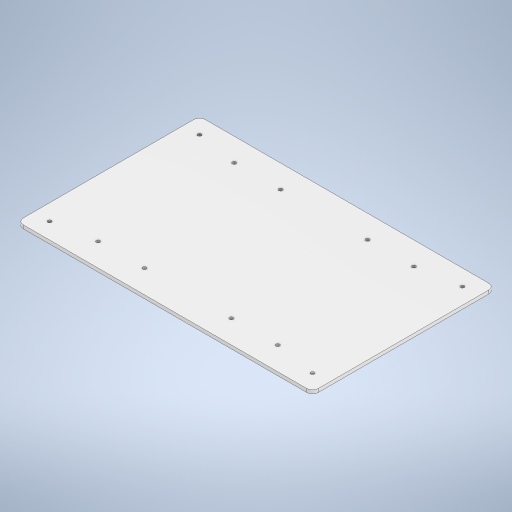
# Autodesk Inventor part: BP_BOX-Under
Saved by Autodesk Inventor 2024.3 (Build 283343000, 343)
## iProperties
Created: 2025-04-29
Part Number: BP_BOX-Under
Material: アセタール樹脂、白
Document SubType Name: Modeling
Designer: ngt-a
Density: 1.425 g/cm^3
Appearance: 滑らか - 白
Mass: 180.144 g
Surface Area: 870.17 cm^2
Volume: 126.417 cm^3
Author: ngt-a
Autodesk Inventor part; units mm, degrees
ref_plane "YZ Plane" through (0, 0, 0) normal (1, 0, 0) x (0, 1, 0)
ref_plane "XZ Plane" through (0, 0, 0) normal (0, 1, 0) x (-1, 0, 0)
ref_plane "XY Plane" through (0, 0, 0) normal (0, 0, 1) x (1, 0, 0)
sketch "スケッチ1" plane through (0, 0, 0) normal (0, 1, 0) x (-1, 0, 0)
  line L0 (130, 81) -> (-130, 81)
  line L1 (-130, 81) -> (-130, -81)
  line L2 (-130, -81) -> (130, -81)
  line L3 (130, -81) -> (130, 81)
  line L4 (130, 81) -> (-130, -81) construction
  line L5 (-130, 81) -> (130, -81) construction
  point P0 (0, 0)
  dimension "d0" = 260
  dimension "d1" = 162
  constraints: 12 end point, 2 midpoint, 2 parallel, 1 horizontal, 1 perpendicular
  measures "d0" distance of L1.end L2.end
  measures "d1" distance of L2.end L0.start
extrude "押し出し1" add sketch "スケッチ1" along normal blind 3
sketch "スケッチ7" plane through (0, 3, 0) normal (0, 1, 0) x (1, 0, 0)
  line L0 (-130, 81) -> (-130, -81) projected
  line L1 (130, -81) -> (130, 81) projected
  line L2 (130, 81) -> (-130, 81) projected
  point P0 (0, 0)
  point P1 (-116, 67)
  point P2 (112, 67)
  point P3 (112, -63)
  point P4 (-116, -63)
  dimension "d23" = 14
  dimension "d25" = 130
  dimension "d26" = 130
  dimension "d27" = 14
  dimension "d29" = 14
  dimension "d38" = 228
  dimension "d39" = 228
  dimension "d40" = 14
  measures "d23" distance from line of L0 point (-116, 67)
  measures "d25" distance of point (112, -63) point (112, 67)
  measures "d26" distance of point (-116, -63) point (-116, 67)
  measures "d27" distance from line of L0 point (-116, -63)
  measures "d29" distance from line of L2 point (-116, 67)
  measures "d38" distance of point (-116, -63) point (112, -63)
  measures "d39" distance of point (-116, 67) point (112, 67)
  measures "d40" distance from line of L2 point (112, 67)
hole "穴1" at (-116, 3, -67) at (112, 3, -67) at (112, 3, 63) at (-116, 3, 63) direction (0, -1, 0) diameter 3.2 depth 8
sketch "スケッチ8" plane through (0, 3, 0) normal (0, 1, 0) x (1, 0, 0)
  line L0 (130, 81) -> (-130, 81) projected
  line L1 (-130, 81) -> (126, 81)
  line L2 (126, 81) -> (126, -77)
  line L3 (126, -77) -> (-130, -77)
  line L4 (-130, -77) -> (-130, 81)
  circle A0 centre (-116, 67) radius 1.6 projected
  circle A1 centre (112, 67) radius 1.6 projected
  circle A2 centre (-116, -63) radius 1.6 projected
  circle A3 centre (-116, -63) radius 1.6 projected
  circle A4 centre (112, -63) radius 1.6 projected
  circle A5 centre (112, 67) radius 1.6 projected
  circle A6 centre (-116, 67) radius 1.6 projected
  line L5 (130, -81) -> (130, 81) projected
  line L6 (130, 81) -> (-130, 81) projected
  line L7 (-130, 81) -> (-130, -81) projected
  line L8 (-130, -81) -> (130, -81) projected
  point P0 (0, 0)
  dimension "d41" = 14
  dimension "d42" = 14
  dimension "d43" = 14
  constraints: 8 end point, 2 parallel, 1 horizontal, 1 perpendicular
  measures "d41" distance from line of L4 A0.centre
  measures "d42" distance from line of L2 A1.centre
  measures "d43" distance from line of L3 A2.centre
extrude "押し出し4" cut sketch "スケッチ8" against normal blind 10 contours L5 L8 L7 L3 L2 L0
fillet "フィレット1" radius 5 4 edges at (-130, 1.5, -81) (-130, 1.5, 77) (126, 1.5, -81) (126, 1.5, 77)
sketch "スケッチ9" plane through (0, 3, 0) normal (0, 1, 0) x (1, 0, 0)
  line L0 (-130, 76) -> (-130, -72) projected
  line L1 (-89.9, 81) -> (-69.9, 81)
  line L2 (-69.8, 81) -> (-49.8, 81)
  line L3 (-49.7, 81) -> (-29.7, 81)
  line L4 (-29.7, -77) -> (-49.7, -77)
  line L5 (0, 0) -> (0, 16.1014)
  circle A0 centre (-116, 67) radius 1.6 projected
  line L6 (126, -72) -> (126, 76) projected
  line L7 (121, 81) -> (-125, 81) projected
  line L8 (-125, -77) -> (121, -77) projected
  line L9 (-69.8, 81) -> (-49.8, 81)
  line L10 (-49.8, 81) -> (-49.8, -77)
  line L11 (-49.8, -77) -> (-69.8, -77)
  line L12 (-69.8, -77) -> (-69.8, 81)
  line L13 (45.8, 81) -> (65.8, 81)
  line L14 (65.8, 81) -> (65.8, -77)
  line L15 (65.8, -77) -> (45.8, -77)
  line L16 (45.8, -77) -> (45.8, 81)
  line L17 (-69.9, 81) -> (-89.9, 81)
  line L18 (-89.9, 81) -> (-89.9, -77)
  line L19 (-89.9, -77) -> (-69.9, -77)
  line L20 (-69.9, -77) -> (-69.9, 81)
  line L21 (121, 81) -> (-125, 81) projected
  line L22 (-49.7, 81) -> (-29.7, 81)
  line L23 (-29.7, 81) -> (-29.7, -77)
  line L24 (-29.7, -77) -> (-49.7, -77)
  line L25 (-49.7, -77) -> (-49.7, 81)
  point P0 (-79.9, 61)
  point P1 (-39.7, 61)
  point P2 (-79.9, -57)
  point P3 (-39.7, -57)
  point P4 (75.9, 61)
  point P5 (35.7, 61)
  point P6 (75.9, -57)
  point P7 (35.7, -57)
  point P8 (-79.9, 81)
  point P9 (-59.8, 61)
  point P10 (55.8, 61)
  point P11 (55.8, -57)
  point P12 (-59.8, -57)
  dimension "d77" = 118
  dimension "d114" = 20
  dimension "d115" = 20
  dimension "d116" = 20
  dimension "d117" = 20
  dimension "d118" = 20
  dimension "d119" = 20
  dimension "d120" = 20
  dimension "d121" = 20
  dimension "d122" = 70.2
  dimension "d123" = 70.2
  dimension "d124" = 20
  dimension "d125" = 70.2
  dimension "d126" = 70.2
  dimension "d127" = 10
  dimension "d128" = 10
  dimension "d129" = 10
  dimension "d130" = 10
  dimension "d131" = 10
  dimension "d132" = 0.1
  dimension "d133" = 50.1
  dimension "d134" = 50.1
  dimension "d135" = 10
  dimension "d136" = 118
  dimension "d137" = 50.1
  dimension "d138" = 10
  dimension "d139" = 0.1
  dimension "d140" = 10
  dimension "d141" = 90.3
  dimension "d142" = 90.3
  dimension "d143" = 90.3
  dimension "d144" = 90.3
  dimension "d145" = 50.1
  constraints: 42 end point, 9 parallel, 7 horizontal, 4 perpendicular, 4 point on line, 1 midpoint, 1 vertical, 5 other
  measures "d77" distance of point (35.7, 61) point (35.7, -57)
  measures "d114" distance of point (-79.9, 81) point (-79.9, 61)
  measures "d116" distance from line of L8 point (-79.9, -57)
  measures "d117" distance from line of L8 point (-39.7, -57)
  measures "d118" distance from line of L8 point (35.7, -57)
  measures "d119" distance from line of L8 point (75.9, -57)
  measures "d122" distance from line of L0 point (-59.8, 61)
  measures "d123" distance from line of L6 point (55.8, 61)
  measures "d124" distance from line of L11 point (-59.8, -57)
  measures "d125" distance from line of L0 point (-59.8, -57)
  measures "d126" distance from line of L6 point (55.8, -57)
  measures "d127" distance from line of L10 point (-59.8, 61)
  measures "d128" distance from line of L12 point (-59.8, 61)
  measures "d129" distance from line of L14 point (55.8, 61)
  measures "d130" distance from line of L16 point (55.8, 61)
  measures "d131" distance from line of L20 point (-79.9, 61)
  measures "d132" distance between parallel lines of L12 L20
  measures "d133" distance from line of L0 point (-79.9, 61)
  measures "d134" distance from line of L6 point (75.9, 61)
  measures "d135" distance from line of L18 point (-79.9, 61)
  measures "d136" distance of point (-79.9, 61) point (-79.9, -57)
  measures "d137" distance from line of L0 point (-79.9, -57)
  measures "d138" distance from line of L25 point (-39.7, -57)
  measures "d139" distance between parallel lines of L10 L25
  measures "d140" distance from line of point (-39.7, -57) L23
  measures "d141" distance from line of L0 point (-39.7, -57)
  measures "d142" distance from line of L0 point (-39.7, 61)
  measures "d143" distance from line of L6 point (35.7, 61)
  measures "d144" distance from line of L6 point (35.7, -57)
  measures "d145" distance from line of L6 point (75.9, -57)
hole "穴2" at (-79.9, 3, -61) at (-39.7, 3, -61) at (-79.9, 3, 57) at (-39.7, 3, 57) at (35.7, 3, 57) at (75.9, 3, 57) at (35.7, 3, -61) at (75.9, 3, -61) direction (0, -1, 0) diameter 3.2 depth 8
sketch "スケッチ12" plane through (0, 0, 0) normal (0, -1, 0) x (1, 0, 0)
  circle A0 centre (75.9, -61) radius 1.6 projected
  circle A1 centre (35.7, -61) radius 1.6 projected
  circle A2 centre (75.9, 57) radius 1.6 projected
  circle A3 centre (35.7, 57) radius 1.6 projected
  circle A4 centre (-39.7, 57) radius 1.6 projected
  circle A5 centre (-79.9, 57) radius 1.6 projected
  circle A6 centre (-39.7, -61) radius 1.6 projected
  circle A7 centre (-79.9, -61) radius 1.6 projected
  arc A8 (126, 72) -> (121, 77) centre (121, 72) ccw projected
  line L0 (121, 77) -> (-125, 77) projected
  arc A9 (-125, 77) -> (-130, 72) centre (-125, 72) ccw projected
  line L1 (-130, -76) -> (-130, 72) projected
  arc A10 (-130, -76) -> (-125, -81) centre (-125, -76) ccw projected
  line L2 (121, -81) -> (-125, -81) projected
  arc A11 (121, -81) -> (126, -76) centre (121, -76) ccw projected
  line L3 (126, -76) -> (126, 72) projected
  circle A12 centre (-116, 63) radius 1.6 projected
  circle A13 centre (112, 63) radius 1.6 projected
  circle A14 centre (112, -67) radius 1.6 projected
  circle A15 centre (-116, -67) radius 1.6 projected
  circle A16 centre (-116, 63) radius 3
  circle A17 centre (-116, -67) radius 3
  circle A18 centre (112, -67) radius 3
  circle A19 centre (112, 63) radius 3
  point P0 (0, 0)
  dimension "d108" = 6
  dimension "d109" = 6
  dimension "d110" = 6
  dimension "d111" = 6
  dimension "d14" = 30
  dimension "d15" = 30
  dimension "d16" = 30
  dimension "d17" = 30
  constraints: 4 centre point
  measures "d108" diameter of A16
  measures "d109" diameter of A17
  measures "d110" diameter of A18
  measures "d111" diameter of A19
extrude "押し出し6" cut sketch "スケッチ12" against normal blind 2 contours A12 | A13 | A14 | A15 | A16 | A17 | A18 | A19
equation "\"d26\" = d25"
equation "\"d27\" = d23"
equation "\"d39\" = d38"
equation "\"d42\" = d41"
equation "\"d43\" = d41"
equation "\"d115\" = d114"
equation "\"d116\" = d114"
equation "\"d117\" = d116"
equation "\"d119\" = d118"
equation "\"d120\" = d118"
equation "\"d121\" = d120"
equation "\"d123\" = d122"
equation "\"d126\" = d123"
equation "\"d129\" = d127"
equation "\"d130\" = d129"
equation "\"d139\" = d132"
equation "\"d140\" = d138"
equation "\"d109\" = d108"
equation "\"d110\" = d109"
equation "\"d111\" = d108"
